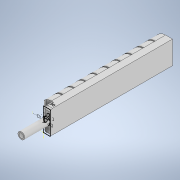
# Autodesk Inventor part: 3D_print_actuator
Saved by Autodesk Inventor 2021 (Build 250183000, 183)
## iProperties
Created: 2021-04-12
Part Number: 3D_print_actuator
Material: Generic
Document SubType Name: Modeling
Designer: Charlie
Density: 1 g/cm^3
Appearance: Default
Author: Charlie
Autodesk Inventor part; units mm, degrees
ref_plane "YZ Plane" through (0, 0, 0) normal (1, 0, 0) x (0, 1, 0)
ref_plane "XY Plane" through (0, 0, 0) normal (0, 0, 1) x (1, 0, 0)
sketch "Sketch1" plane through (0, 0, 0) normal (0, 1, 0) x (-1, 0, 0)
  line L0 (0, 0) -> (0, 100)
  line L1 (0, 0) -> (10.5, 0) construction
  line L2 (15, 4.5) -> (15, 4.5) construction
  line L3 (0, 0) -> (6, 0) construction
  line L4 (10.5, 9) -> (6, 9) construction
  line L5 (6, 9) -> (6, 10)
  line L6 (6, 0) -> (10.5, 0)
  line L7 (15, 9) -> (10.5, 9) construction
  line L8 (15, 9) -> (15, 0) construction
  arc A0 (10.5, 0) -> (15, 4.5) centre (10.5, 4.5) ccw
  arc A1 (15, 4.5) -> (10.5, 9) centre (10.5, 4.5) ccw
  line L9 (10.5, 0) -> (15, 0) construction
  line L10 (10.5, 9) -> (6, 9)
  line L11 (6, 19) -> (6, 20)
  arc A2 (10.5, 10) -> (15, 14.5) centre (10.5, 14.5) ccw
  arc A3 (15, 14.5) -> (10.5, 19) centre (10.5, 14.5) ccw
  line L12 (0, 10) -> (10.5, 10) construction
  line L13 (10.5, 19) -> (6, 19) construction
  line L14 (10.5, 19) -> (6, 19)
  line L15 (6, 10) -> (10.5, 10)
  line L16 (6, 29) -> (6, 30)
  arc A4 (10.5, 20) -> (15, 24.5) centre (10.5, 24.5) ccw
  arc A5 (15, 24.5) -> (10.5, 29) centre (10.5, 24.5) ccw
  line L17 (0, 20) -> (10.5, 20) construction
  line L18 (10.5, 29) -> (6, 29) construction
  line L19 (10.5, 29) -> (6, 29)
  line L20 (6, 20) -> (10.5, 20)
  line L21 (6, 39) -> (6, 40)
  arc A6 (10.5, 30) -> (15, 34.5) centre (10.5, 34.5) ccw
  arc A7 (15, 34.5) -> (10.5, 39) centre (10.5, 34.5) ccw
  line L22 (0, 30) -> (10.5, 30) construction
  line L23 (10.5, 39) -> (6, 39) construction
  line L24 (10.5, 39) -> (6, 39)
  line L25 (6, 30) -> (10.5, 30)
  line L26 (6, 49) -> (6, 50)
  arc A8 (10.5, 40) -> (15, 44.5) centre (10.5, 44.5) ccw
  arc A9 (15, 44.5) -> (10.5, 49) centre (10.5, 44.5) ccw
  line L27 (0, 40) -> (10.5, 40) construction
  line L28 (10.5, 49) -> (6, 49) construction
  line L29 (10.5, 49) -> (6, 49)
  line L30 (6, 40) -> (10.5, 40)
  line L31 (6, 59) -> (6, 60)
  arc A10 (10.5, 50) -> (15, 54.5) centre (10.5, 54.5) ccw
  arc A11 (15, 54.5) -> (10.5, 59) centre (10.5, 54.5) ccw
  line L32 (0, 50) -> (10.5, 50) construction
  line L33 (10.5, 59) -> (6, 59) construction
  line L34 (10.5, 59) -> (6, 59)
  line L35 (6, 50) -> (10.5, 50)
  line L36 (6, 69) -> (6, 70)
  arc A12 (10.5, 60) -> (15, 64.5) centre (10.5, 64.5) ccw
  arc A13 (15, 64.5) -> (10.5, 69) centre (10.5, 64.5) ccw
  line L37 (0, 60) -> (10.5, 60) construction
  line L38 (10.5, 69) -> (6, 69) construction
  line L39 (10.5, 69) -> (6, 69)
  line L40 (6, 60) -> (10.5, 60)
  line L41 (6, 79) -> (6, 80)
  arc A14 (10.5, 70) -> (15, 74.5) centre (10.5, 74.5) ccw
  arc A15 (15, 74.5) -> (10.5, 79) centre (10.5, 74.5) ccw
  line L42 (0, 70) -> (10.5, 70) construction
  line L43 (10.5, 79) -> (6, 79) construction
  line L44 (10.5, 79) -> (6, 79)
  line L45 (6, 70) -> (10.5, 70)
  line L46 (6, 89) -> (6, 90)
  arc A16 (10.5, 80) -> (15, 84.5) centre (10.5, 84.5) ccw
  arc A17 (15, 84.5) -> (10.5, 89) centre (10.5, 84.5) ccw
  line L47 (0, 80) -> (10.5, 80) construction
  line L48 (10.5, 89) -> (6, 89) construction
  line L49 (10.5, 89) -> (6, 89)
  line L50 (6, 80) -> (10.5, 80)
  line L51 (6, 99) -> (6, 100)
  arc A18 (10.5, 90) -> (15, 94.5) centre (10.5, 94.5) ccw
  arc A19 (15, 94.5) -> (10.5, 99) centre (10.5, 94.5) ccw
  line L52 (0, 90) -> (10.5, 90) construction
  line L53 (10.5, 99) -> (6, 99) construction
  line L54 (10.5, 99) -> (6, 99)
  line L55 (6, 90) -> (10.5, 90)
  line L56 (0, 100) -> (0, 106)
  line L57 (0, 106) -> (3, 106)
  line L58 (6, 103) -> (6, 100)
  line L59 (6, 0) -> (0, 0)
  line L60 (6, 103) -> (6, 106)
  line L61 (6, 106) -> (3, 106)
  point P0 (15, 10)
  point P1 (15, 19)
  point P2 (15, 20)
  point P3 (15, 29)
  point P4 (15, 30)
  point P5 (15, 39)
  point P6 (15, 40)
  point P7 (15, 49)
  point P8 (15, 50)
  point P9 (15, 59)
  point P10 (15, 60)
  point P11 (15, 69)
  point P12 (15, 70)
  point P13 (15, 79)
  point P14 (15, 80)
  point P15 (15, 89)
  point P16 (15, 90)
  point P17 (15, 99)
  dimension "d0" = 100
  dimension "d1" = 15
  dimension "d2" = 9
  dimension "d3" = 6
  dimension "d4" = 1
  dimension "d5" = 4.5
  dimension "d6" = 4.5
  dimension "d11" = 10
  dimension "d16" = 6
  dimension "d17" = 6
  dimension "d60" = 99
  dimension "d61" = 30
  dimension "d62" = 30
  dimension "d63" = 30
  constraints: 124 end point, 40 point on circle, 34 point on line, 20 centre point, 5 perpendicular, 5 vertical, 4 collinear, 4 tangent, 3 horizontal, 170 other
  measures "d0" distance of L0.start L0.end
  measures "d1" distance of L0.start L8.end
  measures "d2" distance of L8.end L7.start
  measures "d3" distance of L0.start L3.end
  measures "d4" distance of L4.end L5.end
  measures "d5" radius of A0
  measures "d6" radius of A1
  measures "d11" distance of L4.end L11.start
  measures "d16" distance of L0.end L56.end
  measures "d17" distance of L56.end L60.end
  measures "d60" distance between parallel lines of L6 L53
  measures "d61" distance of A12.centre A18.centre
  measures "d62" distance of A6.centre A12.centre
  measures "d63" distance of A1.centre A6.centre
extrude "Extrusion1" add sketch "Sketch1" along normal blind 20
sketch "Sketch2" plane through (0, 0, 0) normal (0, 0, -1) x (-1, 0, 0)
  line L0 (15, 20) -> (10.5, 20) construction
  line L1 (6, 20) -> (0, 20)
  line L2 (0, 20) -> (0, 0)
  line L3 (0, 0) -> (6, 0)
  line L4 (15, 9) -> (15, 11)
  line L5 (15, 20) -> (0, 0) construction
  arc A0 (15, 11) -> (6, 20) centre (6, 11) ccw
  arc A1 (6, 0) -> (15, 9) centre (6, 9) ccw
  line L6 (-2, -4) -> (17, -4)
  line L7 (17, -4) -> (17, 24)
  line L8 (17, 24) -> (-2, 24)
  line L9 (-2, 24) -> (-2, -4)
  line L10 (-2, -4) -> (17, 24) construction
  line L11 (17, -4) -> (-2, 24) construction
  point P0 (15, 0)
  point P1 (7.5, 10)
  dimension "d21" = 15
  dimension "d22" = 20
  dimension "d23" = 9
  dimension "d24" = 9
  dimension "d25" = 19
  dimension "d26" = 28
  constraints: 22 end point, 4 parallel, 4 point on circle, 4 point on line, 4 tangent, 3 midpoint, 2 centre point, 2 horizontal, 2 perpendicular
  measures "d21" distance of L2.end point (15, 0)
  measures "d22" distance of L1.end L2.end
  measures "d23" radius of A0
  measures "d24" radius of A1
  measures "d25" distance of L8.end L7.end
  measures "d26" distance of L7.end L6.end
extrude "Extrusion2" cut sketch "Sketch2" against normal blind 100
shell "Shell2" thickness 1 removed faces 1 at (-4, 6.6667, 106)
sketch "Sketch7" plane through (-6, 0, 106) normal (0, 0, 1) x (1, 0, 0)
  line L0 (0, 20) -> (6, 20) projected
  line L1 (0, 0) -> (6, 0)
  line L2 (6, 0) -> (6, 20)
  line L3 (6, 20) -> (0, 20)
  line L4 (0, 20) -> (0, 0)
  circle A0 centre (3, 10) radius 0.5 construction
  line L5 (6, 0) -> (6, 20) construction
  line L6 (6, 10) -> (-9, 10) construction
  line L7 (-9, 9) -> (-9, 11) construction
  circle A1 centre (3, 10) radius 3
  circle A2 centre (3, 10) radius 2
  dimension "d46" = 1
  dimension "d80" = 6
  dimension "d81" = 3
  dimension "d82" = 1
  constraints: 10 end point, 3 centre point, 2 midpoint, 2 parallel, 1 horizontal, 1 perpendicular, 1 point on line
  measures "d46" diameter of A0
  measures "d80" diameter of A1
  measures "d81" distance from line of L2 A1.centre
  measures "d82" radial gap between concentric circles of A1 A2
extrude "Extrusion5" add sketch "Sketch7" against normal blind 8 contours L0 L2 A1 L4 | A1 L2 L1 L4 | A1 | A2
fillet "Fillet2" radius 2 5 edges at (-6, 20, 102.5) (-6, 10, 106) (-6, 0, 102.5) (-3, 0, 106) (-3, 20, 106)
sketch "Sketch8" plane through (0, 0, 0) normal (1, 0, 0) x (0, 1, 0)
  line L0 (0, 9) -> (20, 9) projected
  line L1 (0, 10) -> (20, 10) projected
  line L2 (0, 9) -> (20, 9)
  line L3 (20, 9) -> (20, 10)
  line L4 (20, 10) -> (0, 10)
  line L5 (0, 10) -> (0, 9)
  line L6 (0, 19) -> (20, 19)
  line L7 (20, 20) -> (0, 20)
  line L8 (20, 19) -> (20, 20)
  line L9 (0, 20) -> (0, 19)
  line L10 (0, 29) -> (20, 29)
  line L11 (20, 30) -> (0, 30)
  line L12 (20, 29) -> (20, 30)
  line L13 (0, 30) -> (0, 29)
  line L14 (0, 39) -> (20, 39)
  line L15 (20, 40) -> (0, 40)
  line L16 (20, 39) -> (20, 40)
  line L17 (0, 40) -> (0, 39)
  line L18 (0, 49) -> (20, 49)
  line L19 (20, 50) -> (0, 50)
  line L20 (20, 49) -> (20, 50)
  line L21 (0, 50) -> (0, 49)
  line L22 (0, 59) -> (20, 59)
  line L23 (20, 60) -> (0, 60)
  line L24 (20, 59) -> (20, 60)
  line L25 (0, 60) -> (0, 59)
  line L26 (0, 69) -> (20, 69)
  line L27 (20, 70) -> (0, 70)
  line L28 (20, 69) -> (20, 70)
  line L29 (0, 70) -> (0, 69)
  line L30 (0, 79) -> (20, 79)
  line L31 (20, 80) -> (0, 80)
  line L32 (20, 79) -> (20, 80)
  line L33 (0, 80) -> (0, 79)
  line L34 (0, 89) -> (20, 89)
  line L35 (20, 90) -> (0, 90)
  line L36 (20, 89) -> (20, 90)
  line L37 (0, 90) -> (0, 89)
  point P0 (0, 0)
  dimension "d51" = 10
  constraints: 72 end point, 2 parallel, 1 collinear, 1 horizontal, 1 perpendicular, 1 vertical, 63 other
  measures "d51" distance of L0.start L6.start
extrude "Extrusion7" add sketch "Sketch8" against normal blind 6
ref_plane "Work Plane1" through (-6, 0, 99) normal (0, 0, 1) x (1, 0, 0)
sketch "Sketch4" plane through (-6, 0, 99) normal (0, 0, 1) x (1, 0, 0)
  line L0 (0, 0) -> (0, 20) projected
  line L1 (0, 0) -> (6, 20) construction
  circle A0 centre (3, 10) radius 2
  line L2 (5, 6.5) -> (1, 6.5)
  line L3 (1, 6.5) -> (1, 13.5)
  line L4 (1, 13.5) -> (5, 13.5)
  line L5 (5, 13.5) -> (5, 6.5)
  line L6 (5, 6.5) -> (1, 13.5) construction
  line L7 (1, 6.5) -> (5, 13.5) construction
  point P0 (6, 0)
  point P1 (3, 10)
  point P2 (1, 10)
  point P3 (5, 10)
  dimension "d31" = 4
  dimension "d58" = 4
  dimension "d59" = 7
  constraints: 14 end point, 3 midpoint, 2 parallel, 1 centre point, 1 horizontal, 1 perpendicular
  measures "d31" diameter of A0
  measures "d58" distance of L3.end L4.end
  measures "d59" distance of L2.end L3.end
extrude "Extrusion3" cut sketch "Sketch4" against normal blind 96 contours A0
sketch "Sketch9" plane through (-10.5, 1.2058, 99) normal (0, 0, 1) x (1, 0, 0)
  line L0 (-4.5, 7.7942) -> (-4.5, 9.7942) construction
  line L1 (-4.5, 8.7942) -> (0.5, 8.7942) construction
  line L2 (0, 1.1799) -> (0, 16.4086) construction
  circle A0 centre (0.5, 8.7942) radius 0.125
  point P0 (10.5, -1.2058)
  dimension "d64" = 5
  dimension "d65" = 0.25
  constraints: 2 end point, 1 centre point, 1 coincident, 1 midpoint, 1 perpendicular
  measures "d64" distance of L1.start L1.end
  measures "d65" diameter of A0
sketch "Sketch10" plane through (-6, 0, 69) normal (0, 0, 1) x (1, 0, 0)
  line L0 (-9, 9) -> (-9, 11) construction
  line L1 (-9, 10) -> (-4, 10) construction
  circle A0 centre (-4, 10) radius 0.125
  point P0 (6, 0)
  dimension "d66" = 5
  dimension "d67" = 0.25
  constraints: 2 end point, 1 centre point, 1 coincident, 1 horizontal, 1 midpoint
  measures "d66" distance of L1.start L1.end
  measures "d67" diameter of A0
sketch "Sketch11" plane through (-6, 0, 39) normal (0, 0, 1) x (1, 0, 0)
  line L0 (-9, 9) -> (-9, 11) construction
  line L1 (-9, 10) -> (-4, 10) construction
  circle A0 centre (-4, 10) radius 0.125
  point P0 (6, 0)
  dimension "d68" = 5
  dimension "d69" = 0.25
  constraints: 2 end point, 1 centre point, 1 coincident, 1 horizontal, 1 midpoint
  measures "d68" distance of L1.start L1.end
  measures "d69" diameter of A0
sketch "Sketch12" plane through (-6, 0, 9) normal (0, 0, 1) x (1, 0, 0)
  line L0 (-9, 9) -> (-9, 11) construction
  line L1 (-9, 10) -> (-4, 10) construction
  circle A0 centre (-4, 10) radius 0.125
  point P0 (6, 0)
  dimension "d70" = 5
  dimension "d71" = 0.25
  constraints: 2 end point, 1 centre point, 1 coincident, 1 horizontal, 1 midpoint
  measures "d70" distance of L1.start L1.end
  measures "d71" diameter of A0
extrude "Extrusion8" cut sketch "Sketch9" against normal blind 9
extrude "Extrusion9" cut sketch "Sketch10" against normal blind 9
extrude "Extrusion10" cut sketch "Sketch11" against normal blind 9
extrude "Extrusion11" cut sketch "Sketch12" against normal blind 9
extrude "Extrusion12" add sketch "Sketch7" along normal blind 22 and the other way blind 7 contours A1
extrude "Extrusion13" cut sketch "Sketch7" against normal blind 12 contours A2
sketch "version number" plane through (0, 20, 0) normal (0, 1, 0) x (1, 0, 0)
  line L0 (-4.1964, -102.3307) -> (-4.1964, -100.0435) construction
  line L1 (-4.1964, -100.0435) -> (-1.1484, -100.0435) construction
  line L2 (-1.1484, -100.0435) -> (-1.1484, -102.3307) construction
  line L3 (-1.1484, -102.3307) -> (-4.1964, -102.3307) construction
  spline S0 degree 2 poles (-1.0101, -101.1871) (-1.0101, -101.4143) (-1.146, -101.7873) (-1.2719, -101.9182) knots 0 0 0 1 2 2 2
  spline S1 degree 2 poles (-1.2719, -101.9182) (-1.3954, -102.0466) (-1.7314, -102.18) (-1.9216, -102.18) knots 0 0 0 1 2 2 2
  spline S2 degree 2 poles (-1.9216, -102.18) (-2.1686, -102.18) (-2.5835, -101.9157) (-2.707, -101.6638) knots 0 0 0 1 2 2 2
  line L4 (-2.707, -101.6638) -> (-2.7194, -101.6638)
  spline S3 degree 2 poles (-2.7194, -101.6638) (-2.8503, -101.8886) (-3.1615, -102.1059) (-3.3937, -102.1059) knots 0 0 0 1 2 2 2
  spline S4 degree 2 poles (-3.3937, -102.1059) (-3.737, -102.1059) (-4.1964, -101.5872) (-4.1964, -101.1871) knots 0 0 0 1 2 2 2
  spline S5 degree 2 poles (-4.1964, -101.1871) (-4.1964, -100.7721) (-3.7617, -100.2707) (-3.4208, -100.2707) knots 0 0 0 1 2 2 2
  spline S6 degree 2 poles (-3.4208, -100.2707) (-3.2158, -100.2707) (-2.8157, -100.5103) (-2.7021, -100.7351) knots 0 0 0 1 2 2 2
  line L5 (-2.7021, -100.7351) -> (-2.6897, -100.7351)
  spline S7 degree 2 poles (-2.6897, -100.7351) (-2.5662, -100.4683) (-2.2105, -100.1941) (-1.929, -100.1941) knots 0 0 0 1 2 2 2
  spline S8 degree 2 poles (-1.929, -100.1941) (-1.5387, -100.1941) (-1.0101, -100.7622) (-1.0101, -101.1871) knots 0 0 0 1 2 2 2
  spline S9 degree 2 poles (-1.8894, -100.614) (-2.0772, -100.614) (-2.2995, -100.7622) (-2.4131, -100.9722) knots 0 0 0 1 2 2 2
  spline S10 degree 2 poles (-2.4131, -100.9722) (-2.4526, -101.0413) (-2.544, -101.2735) (-2.6033, -101.4193) knots 0 0 0 1 2 2 2
  spline S11 degree 2 poles (-2.6033, -101.4193) (-2.4921, -101.5872) (-2.1611, -101.7675) (-1.9512, -101.7675) knots 0 0 0 1 2 2 2
  spline S12 degree 2 poles (-1.9512, -101.7675) (-1.6745, -101.7675) (-1.3139, -101.4341) (-1.3139, -101.1821) knots 0 0 0 1 2 2 2
  spline S13 degree 2 poles (-1.3139, -101.1821) (-1.3139, -100.9252) (-1.6227, -100.614) (-1.8894, -100.614) knots 0 0 0 1 2 2 2
  spline S14 degree 2 poles (-3.4159, -100.6708) (-3.6209, -100.6708) (-3.8951, -100.945) (-3.8951, -101.1895) knots 0 0 0 1 2 2 2
  spline S15 degree 2 poles (-3.8951, -101.1895) (-3.8951, -101.4118) (-3.6506, -101.6959) (-3.4406, -101.6959) knots 0 0 0 1 2 2 2
  spline S16 degree 2 poles (-3.4406, -101.6959) (-3.2899, -101.6959) (-3.08, -101.5502) (-2.996, -101.4044) knots 0 0 0 1 2 2 2
  spline S17 degree 2 poles (-2.996, -101.4044) (-2.9614, -101.3427) (-2.8404, -101.0809) (-2.8058, -100.9746) knots 0 0 0 1 2 2 2
  spline S18 degree 2 poles (-2.8058, -100.9746) (-2.9417, -100.7968) (-3.2307, -100.6708) (-3.4159, -100.6708) knots 0 0 0 1 2 2 2
  point P0 (0, 0)
  constraints: 2 other
extrude "Extrusion14" cut sketch "version number" against normal blind 0.5
sketch "Sketch6" plane through (0, 10, 0) normal (0, 1, 0) x (-1, 0, 0)
  line L0 (21.0864, 109.726) -> (-9.863, 109.726)
  line L1 (-9.863, 109.726) -> (-9.863, -3.5286)
  line L2 (-9.863, -3.5286) -> (21.0864, -3.5286)
  line L3 (21.0864, -3.5286) -> (21.0864, 109.726)
  point P0 (0, 0)
  dimension "d36" = 113.2546
  dimension "d37" = 30.9494
  constraints: 8 end point, 2 parallel, 1 horizontal, 1 perpendicular
  measures "d36" distance of L2.end L0.start
  measures "d37" distance of L1.end L2.end
body "Solid1"
